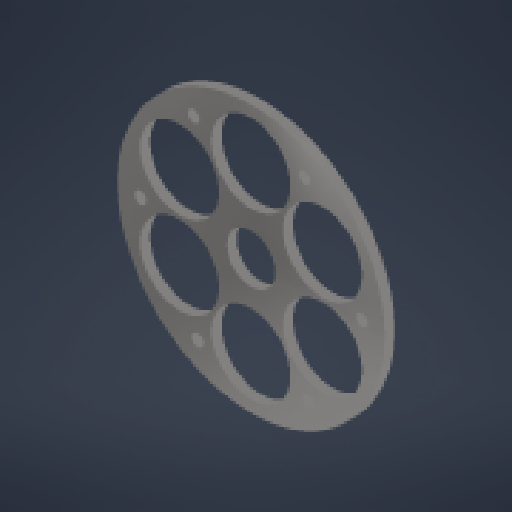
# Autodesk Inventor part: Electromagnetic cover bottom
Saved by Autodesk Inventor 2026.3 (Build 303398000, 398)
## iProperties
Created: 2026-08-03
Part Number: Electromagnetic cover bottom
Material: Generic
Document SubType Name: Sheet Metal
Designer: matot
Density: 1 g/cm^3
Sheet Metal Rule: Default_mm
Appearance: Default
Author: matot
Autodesk Inventor part; units mm, degrees
ref_plane "YZ Plane" through (0, 0, 0) normal (1, 0, 0) x (0, 1, 0)
ref_plane "XZ Plane" through (0, 0, 0) normal (0, 1, 0) x (-1, 0, 0)
ref_plane "XY Plane" through (0, 0, 0) normal (0, 0, 1) x (1, 0, 0)
sketch "Sketch1" plane through (0, 0, 0) normal (0, 0, 1) x (1, 0, 0)
  circle A0 centre (0, 0) radius 55
  circle A1 centre (0, 0) radius 10
  dimension "d0" = 110
  dimension "d1" = 20
  constraints: 2 centre point, 2 coincident
  measures "d0" diameter of A0
  measures "d1" diameter of A1
extrude "Extrusion1" add sketch "Sketch1" along normal blind 4
sketch "Sketch2" plane through (0, 0, 4) normal (0, 0, 1) x (1, 0, 0)
  point P0 (0, 0)
  point P1 (0, 34)
  point P2 (-29.4449, 17)
  point P3 (-29.4449, -17)
  point P4 (0, -34)
  point P5 (29.4449, -17)
  point P6 (29.4449, 17)
  dimension "d4" = 34
  dimension "d7" = 360
  constraints: 7 other
  measures "d4" distance of point (0, 34) point (0, 0)
hole "Hole1" at (0, 34, 4) at (-29.4449, 17, 4) at (-29.4449, -17, 4) at (0, -34, 4) at (29.4449, -17, 4) at (29.4449, 17, 4) direction (0, 0, -1) diameter 32.5 end through all
sketch "Sketch3" plane through (0, 0, 4) normal (0, 0, 1) x (1, 0, 0)
  point P0 (0, 0)
  point P1 (22, 40)
  point P2 (-23.641, 39.0526)
  point P3 (-45.641, -0.9474)
  point P4 (-22, -40)
  point P5 (23.641, -39.0526)
  point P6 (45.641, 0.9474)
  dimension "d18" = 360
  constraints: 7 other
hole "Hole2" at (22, 40, 4) at (-23.641, 39.0526, 4) at (-45.641, -0.9474, 4) at (-22, -40, 4) at (23.641, -39.0526, 4) at (45.641, 0.9474, 4) direction (0, 0, -1) diameter 5 end through all
equation "\"d14\" = Thickness"
equation "\"BendRadius\" = Thickness"
equation "\"BendReliefWidth\" = Thickness"
equation "\"BendReliefDepth\" = 0.5 * Thickness"
equation "\"CornerReliefSize\" = 4 * Thickness"
equation "\"MinimumRemnant\" = 2 * Thickness"
equation "\"TransitionRadius\" = BendRadius"
equation "\"JacobiRadiusSize\" = BendRadius"
equation "\"GapSize\" = Thickness"
equation "\"Thickness\" = 0.5"
body "Solid1"
